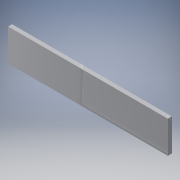
# Autodesk Inventor part: supportbeam2
Saved by Autodesk Inventor 2016 (Build 200138000, 138)
## iProperties
Created: 2016-01-29
Part Number: supportbeam2
Material: Aluminum 6061
Document SubType Name: Modeling
Designer: zachary
Density: 2.7 g/cm^3
Appearance: Aluminum - Flat
Mass: 26.9019 g
Surface Area: 73.7464 cm^2
Volume: 9.96368 cm^3
User Status: in process
Author: zachary
Autodesk Inventor part; units mm, degrees
ref_plane "YZ Plane" through (0, 0, 0) normal (1, 0, 0) x (0, 1, 0)
ref_plane "XZ Plane" through (0, 0, 0) normal (0, 1, 0) x (-1, 0, 0)
ref_plane "XY Plane" through (0, 0, 0) normal (0, 0, 1) x (1, 0, 0)
sketch "Sketch1" plane through (0, 0, 0) normal (0, 0, 1) x (1, 0, 0)
  line L0 (0, 0) -> (-126.365, 0)
  line L1 (-126.365, 0) -> (-126.365, -25.4)
  line L2 (-126.365, -25.4) -> (0, -25.4)
  line L3 (0, -25.4) -> (0, 0)
  dimension "d0" = 126.365
  dimension "d1" = 25.4
  constraints: 8 end point, 2 parallel, 1 horizontal, 1 perpendicular
  measures "d0" distance between parallel lines of L1 L3
  measures "d1" distance between parallel lines of L0 L2
extrude "Extrusion1" add sketch "Sketch1" along normal blind 3.175
sketch "Sketch2" plane through (0, 0, 0) normal (0, 0, -1) x (-1, 0, 0)
  circle A0 centre (38.1, -12.7) radius 3.3734
  circle A1 centre (12.7, -12.7) radius 3.3734
  line L0 (0, 0) -> (126.365, 0) projected
  line L1 (0, -25.4) -> (0, 0) projected
  dimension "d4" = 6.7469
  dimension "d5" = 12.7
  dimension "d6" = 12.7
  dimension "d7" = 25.4
  dimension "d8" = 12.7
  constraints: 2 centre point, 1 equal radius
  measures "d4" diameter of A0
  measures "d5" distance from line of L0 A1.centre
  measures "d6" distance from line of L1 A1.centre
  measures "d7" distance of A0.centre A1.centre
  measures "d8" distance from line of L0 A0.centre
extrude "Extrusion2" cut sketch "Sketch2" against normal blind 3.175
body "Solid1"
